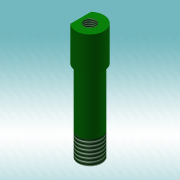
# Autodesk Inventor part: 回転アーム付き計測輪シャフト
Saved by Autodesk Inventor 2015 (Build 190159000, 159)
## iProperties
Created: 2016-04-01
Part Number: 回転アーム付き計測輪シャフト
Material: 一般
Document SubType Name: Modeling
Designer: buzztaka
Density: 1 g/cm^3
Appearance: 濃い緑
Author: buzztaka
Autodesk Inventor part; units mm, degrees
ref_plane "YZ Plane" through (0, 0, 0) normal (1, 0, 0) x (0, 1, 0)
ref_plane "XZ Plane" through (0, 0, 0) normal (0, 1, 0) x (-1, 0, 0)
sketch "スケッチ1" plane through (0, 0, 0) normal (0, 0, 1) x (1, 0, 0)
  point P0 (0, 0)
sketch "スケッチ2" plane through (0, 0, 0) normal (0, 0, 1) x (1, 0, 0)
  circle A0 centre (0, 0) radius 5
  dimension "d0" = 10
  constraints: 1 centre point, 1 coincident
  measures "d0" diameter of A0
extrude "押し出し1" add sketch "スケッチ2" along normal blind 35
thread "ねじ1" size "M10x1.5" class "6g" standard "ANSI Metric M Profile" length 10
sketch "スケッチ3" plane through (0, 0, 35) normal (0, 0, 1) x (1, 0, 0)
  point P0 (0, 0)
sketch "スケッチ4" plane through (0, 0, 35) normal (0, 0, 1) x (1, 0, 0)
  circle A0 centre (0, 0) radius 6
  dimension "d5" = 12
  constraints: 1 centre point, 1 coincident
  measures "d5" diameter of A0
extrude "押し出し2" add sketch "スケッチ4" along normal blind 14.85
sketch "スケッチ5" plane through (0, 0, 49.85) normal (0, 0, 1) x (1, 0, 0)
  line L0 (0, 0) -> (0, 6)
  circle A0 centre (0, 0) radius 6 projected
  constraints: 2 end point, 1 vertical alignment, 1 other
ref_plane "作業平面1" through (0, 6, 49.85) normal (0, 1, 0) x (-1, 0, 0)
sketch "スケッチ9" plane through (0, 0, 49.85) normal (0, 0, 1) x (1, 0, 0)
  point P0 (0, 0)
  point P1 (0, 0)
  constraints: 1 coincident
hole "穴2" at (0, 0, 49.85) direction (0, 0, -1) diameter 5 depth 8 tip angle 118
thread "ねじ3" size "M5x0.8" class "6H" standard "ANSI Metric M Profile" full length
sketch "スケッチ10" plane through (0, 0, 49.85) normal (0, 0, 1) x (1, 0, 0)
  arc A0 (-4, 4.4721) -> (-4, -4.4721) centre (0, 0) ccw
  line L0 (-4, 0) -> (-4, 4.4721)
  line L1 (-4, 0) -> (-4, -4.4721)
  dimension "d34" = 12
  dimension "d35" = 4
  constraints: 4 end point, 2 point on circle, 1 centre point, 1 coincident, 1 point on line, 1 vertical
  measures "d34" diameter of A0
  measures "d35" distance of L0.start point (0, 0)
extrude "押し出し4" cut sketch "スケッチ10" against normal blind 5
